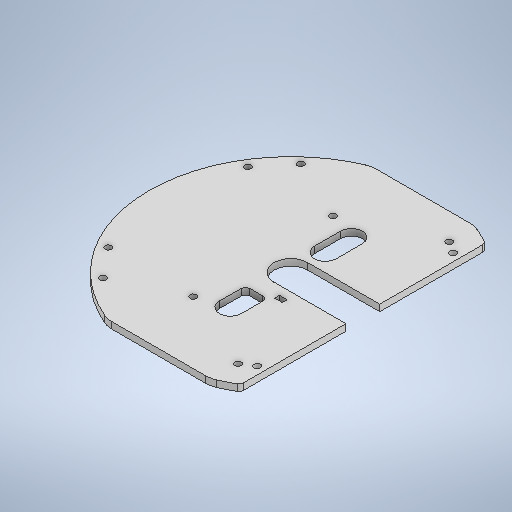
# Autodesk Inventor part: base_nivel2
Saved by Autodesk Inventor 2025.2 (Build 292293000, 293)
## iProperties
Created: 2025-04-02
Part Number: base_nivel2
Material: Generic
Document SubType Name: Modeling
Designer: cdavi
Density: 1 g/cm^3
Appearance: Default
Author: cdavi
Autodesk Inventor part; units mm, degrees
ref_plane "YZ Plane" through (0, 0, 0) normal (1, 0, 0) x (0, 1, 0)
ref_plane "XZ Plane" through (0, 0, 0) normal (0, 1, 0) x (-1, 0, 0)
ref_plane "XY Plane" through (0, 0, 0) normal (0, 0, 1) x (1, 0, 0)
sketch "Sketch1" plane through (0, 0, 0) normal (0, 1, 0) x (-1, 0, 0)
  circle A0 centre (0, 0) radius 53.7304
  line L0 (0, 53.7304) -> (0, -53.7304)
  circle A1 centre (-29.5, 44.9077) radius 1.5
  line L1 (0, 0) -> (-53.7304, 0)
  circle A2 centre (-29.5, -44.9077) radius 1.5
  line L2 (-33, 56) -> (-33, -56)
  circle A3 centre (0, 0) radius 7.75
  line L3 (0, 7.75) -> (-33, 7.75)
  line L4 (0, -7.75) -> (-33, -7.75)
  circle A4 centre (0, 0) radius 65
  circle A5 centre (-29.5, -44.9077) radius 1.5
  line L5 (12.75, 32) -> (51.75, 32)
  line L6 (51.75, 32) -> (51.75, -32)
  line L7 (51.75, -32) -> (12.75, -32) construction
  line L8 (12.75, -32) -> (12.75, 32)
  circle A6 centre (0, 0) radius 70 construction
  line L9 (-40, 57.4456) -> (-40, -57.4456)
  line L10 (0, 0) -> (-29.5, 44.9077) construction
  circle A7 centre (-24.2, 48.4456) radius 1.5
  circle A8 centre (-24.2, -48.4456) radius 1.5
  circle A9 centre (51.75, -32) radius 1.5
  line L11 (51.75, -32) -> (55.2843, -34.1855)
  circle A10 centre (51.75, 32) radius 1.5
  circle A11 centre (12.75, 32) radius 1.5
  circle A12 centre (12.75, -32) radius 1.5
  circle A13 centre (40.817, 45.3318) radius 1.5
  circle A14 centre (40.817, -45.3318) radius 1.5
  line L12 (-6.5, 11.75) -> (-10, 11.75)
  line L13 (-10, 11.75) -> (-10, 13.95)
  line L14 (-10, 13.95) -> (-6.5, 13.95)
  line L15 (-6.5, 13.95) -> (-6.5, 11.75)
  line L16 (0, 27.8) -> (0, 15.8) construction
  line L17 (-5, 27.8) -> (-5, 15.8)
  line L18 (5, 15.8) -> (5, 27.8)
  arc A15 (5, 27.8) -> (-5, 27.8) centre (0, 27.8) ccw
  arc A16 (-5, 15.8) -> (5, 15.8) centre (0, 15.8) ccw
  line L19 (-5, -27.8) -> (-5, -15.8)
  line L20 (5, -15.8) -> (5, -27.8)
  arc A17 (-5, -27.8) -> (5, -27.8) centre (0, -27.8) ccw
  arc A18 (5, -15.8) -> (-5, -15.8) centre (0, -15.8) ccw
  line L21 (5, 15.8) -> (-5, 15.8)
  line L22 (0, 0) -> (-12.842, 0) construction
  line L23 (-10, 11.75) -> (-26.65, 11.75) construction
  line L24 (-26.65, 11.75) -> (-26.65, 0) construction
  line L25 (-26.65, 0) -> (-17.65, 0)
  line L26 (23.5, -60.6032) -> (23.5, 60.6032) construction
  line L27 (23.5, -60.6032) -> (-23.5, -60.6032)
  line L28 (23.5, 60.6032) -> (-23.5, 60.6032)
  line L29 (0, 0) -> (40.817, 45.3318)
  point P0 (12.75, 0)
  point P1 (7.75, 0)
  point P2 (0, -7.75)
  point P3 (51.75, -14.4531)
  point P4 (51.75, -30.5)
  point P5 (50.25, -32)
  point P6 (43.1619, -32)
  point P7 (51.75, 14.4531)
  point P8 (43.1619, 32)
  point P9 (50.25, 32)
  point P10 (51.75, 30.5)
  point P11 (0, 21.8)
  point P12 (0, 10.8)
  point P13 (0, 32.8)
  point P14 (-40, -51.2348)
  point P15 (-40, 51.2348)
  point P16 (52.6522, 30.8017)
  point P17 (51.081, 33.3426)
  point P18 (51.081, -33.3426)
  point P19 (52.6522, -30.8017)
  dimension "d5" = 130
  dimension "d2" = 3
  dimension "d3" = 33
  dimension "d4" = 15.5
  dimension "d6" = 39
  dimension "d7" = 64
  dimension "d8" = 5
  dimension "d9" = 140
  dimension "d11" = 40
  dimension "d15" = 107.4608
  dimension "d16" = 33.301
  dimension "d17" = 3
  dimension "d18" = 15.8
  dimension "d19" = 9
  dimension "d20" = 3
  dimension "d21" = 4.1554
  dimension "d40" = 2.2
  dimension "d41" = 3.5
  dimension "d42" = 4
  dimension "d43" = 23
  dimension "d45" = 10
  dimension "d46" = 22
  dimension "d49" = 21.8
  dimension "d51" = 12.842
  dimension "d52" = 16.65
  dimension "d53" = 9
  dimension "d54" = 4.808
  dimension "d56" = 3.3723
  dimension "d57" = 23.5
  dimension "d58" = 42
  dimension "d59" = 61
  dimension "d60" = 3
  constraints: 62 end point, 18 centre point, 18 point on circle, 11 symmetric about line, 9 coincident, 7 point on line, 6 horizontal, 5 parallel, 5 perpendicular, 5 tangent, 4 midpoint, 4 vertical, 3 equal radius, 2 horizontal alignment, 16 other
  measures "d2" diameter of A1
  measures "d3" distance between parallel lines of L0 L2
  measures "d4" diameter of A3
  measures "d6" distance between parallel lines of L8 L6
  measures "d7" distance of L5.end L6.end
  measures "d8" distance from line of A3.end L8
  measures "d9" diameter of A6
  measures "d11" distance from line of L9 A3.centre
  measures "d15" diameter of A0
  measures "d16" angle of L0 L10
  measures "d17" diameter of A7
  measures "d18" horizontal distance of L9.start A7.centre
  measures "d19" vertical distance of L9.start A7.centre
  measures "d20" diameter of A9
  measures "d21" distance of L11.start L11.end
  measures "d40" distance of L14.end L12.start
  measures "d41" distance of L13.end L14.end
  measures "d42" distance between parallel lines of L3 L12
  measures "d43" distance between parallel lines of L2 L13
  measures "d45" distance between parallel lines of L17 L18
  measures "d46" distance of point (0, 10.8) point (0, 32.8)
  measures "d49" distance of point (0, 0) point (0, 21.8)
  measures "d51" distance of point (0, 0) L22.end
  measures "d52" distance of L12.end L23.end
  measures "d53" distance of L24.end L25.end
  measures "d54" distance of L25.end L22.end
  measures "d57" distance from line of point (0, 0) L26
  measures "d58" angle of L0 L29
  measures "d59" distance of L22.start L29.end
  measures "d60" diameter of A13
extrude "Extrusion1" add sketch "Sketch1" along normal blind 3 contours A0 L6 | A0 L6 A10 L5 A7 A1 L2 A4 L28 L11 A9 | L6 A0 L0 A17 L20 A18 A3 L29 L5 | A0 L5 A10 L6 | L6 A9 L11 A4 L27 L2 A0 A2 A8 | L5 L29 A0 | A0 A8 A2 L2 L4 L0 A18 L19 A17 | L29 L5 A11 L8 A3 L0 A16 L18 A15 A0 | L29 L8 A11 L5 | L0 A15 L17 A16 L3 L2 A0 A1 A7 | L21 A16 L0 | L0 A16 L21
fillet "Fillet1" radius 2 4 edges at (-5, 1.5, 15.8) (5, 1.5, 15.8) (33, 1.5, 56) (33, 1.5, -56)
fillet "Fillet2" radius 10 4 edges at (23.5, 1.5, 60.6032) (-23.5, 1.5, 60.6032) (23.5, 1.5, -60.6032) (-23.5, 1.5, -60.6032)
body "Solid1"
